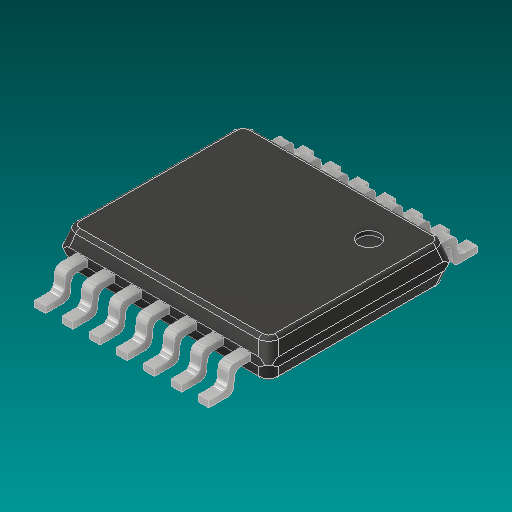
# Autodesk Inventor part: TSSOP
Saved by Autodesk Inventor 2017 (Build 210142000, 142)
## iProperties
Created: 2016-07-25
Part Number: TSSOP
Material: Generic
Document SubType Name: Modeling
Designer: Jonathan
Density: 1 g/cm^3
Appearance: Default
Author: Jonathan
Autodesk Inventor part; units mm, degrees
ref_plane "YZ Plane" through (0, 0, 0) normal (1, 0, 0) x (0, 1, 0)
ref_plane "XZ Plane" through (0, 0, 0) normal (0, 1, 0) x (-1, 0, 0)
ref_plane "XY Plane" through (0, 0, 0) normal (0, 0, 1) x (1, 0, 0)
sketch "Sketch1" plane through (0, 0, 0) normal (0, 1, 0) x (-1, 0, 0)
  line L0 (2.5, 2.2) -> (-2.5, 2.2)
  line L1 (-2.5, 2.2) -> (-2.5, -2.2)
  line L2 (-2.5, -2.2) -> (2.5, -2.2)
  line L3 (2.5, -2.2) -> (2.5, 2.2)
  line L4 (2.5, 2.2) -> (-2.5, -2.2) construction
  line L5 (-2.5, 2.2) -> (2.5, -2.2) construction
  point P0 (0, 0)
  dimension "d0" = 5
  dimension "d1" = 4.4
  constraints: 12 end point, 2 midpoint, 2 parallel, 1 horizontal, 1 perpendicular
  measures "d0" distance of L1.end L2.end
  measures "d1" distance of L0.end L1.end
extrude "Extrusion1" add sketch "Sketch1" along normal blind 0.9
sketch "Sketch3" plane through (0, 0, 0) normal (1, 0, 0) x (0, 1, 0)
  line L0 (0, 2.2) -> (0.9, 2.2) projected
  line L1 (0.525, 2.2) -> (0.525, 2.7167)
  line L2 (0.525, 2.7167) -> (0.05, 2.7582)
  line L3 (0.05, 2.7582) -> (0.05, 3.2)
  line L4 (0.05, 3.2) -> (-0.1, 3.2)
  line L5 (-0.1, 3.2) -> (-0.1, 2.6208)
  line L6 (-0.1, 2.6208) -> (0.375, 2.5792)
  line L7 (0.375, 2.5792) -> (0.375, 2.2)
  line L8 (0.525, 2.2) -> (0.375, 2.2)
  line L9 (0, 2.2) -> (0, -2.2) projected
  point P0 (0, 0)
  point P1 (0.1375, 2.6)
  point P2 (0.45, 2.2)
  dimension "d4" = 0.15
  dimension "d5" = 0.15
  dimension "d6" = 0.15
  dimension "d7" = 0.6
  dimension "d8" = 3.2
  dimension "d10" = 0.1
  dimension "d11" = 95
  constraints: 16 end point, 3 midpoint, 3 parallel, 2 perpendicular, 2 point on line, 1 collinear, 1 vertical
  measures "d4" distance between parallel lines of L5 L3
  measures "d5" distance between parallel lines of L2 L6
  measures "d6" distance between parallel lines of L1 L7
  measures "d7" distance from line of L4 point (0.138, 2.6)
  measures "d8" distance from line of point (0, 0) L4
  measures "d10" distance between parallel lines of L5 L9
  measures "d11" angle of L6 L5
extrude "Extrusion2" add sketch "Sketch3" along normal mid plane 0.25 separate body
fillet "Fillet1" radius 0.15 4 edges at (0, 0.05, 2.7582) (0, 0.525, 2.7167) (0, 0.375, 2.5792) (0, -0.1, 2.6208)
pattern_linear "Rectangular Pattern1" count 4 spacing 0.65 along (1, 0, 0) count 4 spacing 0.65 along (-1, 0, 0) of "Extrusion2", "Fillet1" bodies 2
mirror "Mirror1" about plane through (0, 0, 0) normal (0, 0, 1) of "Extrusion2", "Fillet1", "Rectangular Pattern1" bodies 2
chamfer "Chamfer1" distance 0.1 distance2 0.35 1 edges at (0, 0.9, 2.2) measured on face at (0.8333, 0.9, -0.7333)
chamfer "Chamfer2" distance 0.1 distance2 0.35 1 edges at (0, 0.9, -2.2) measured on face at (0.8333, 0.9, -0.7667)
chamfer "Chamfer3" distance 0.1 distance2 0.35 1 edges at (2.5, 0.9, 0) measured on face at (0.8333, 0.9, -0.7)
chamfer "Chamfer4" distance 0.1 distance2 0.35 1 edges at (-2.5, 0.9, 0) measured on face at (-0.8667, 0.9, -0.7)
chamfer "Chamfer5" distance 0.35 distance2 0.1 1 edges at (0, 0, 2.2) measured on face at (0.8333, 0.3667, 2.2)
chamfer "Chamfer6" distance 0.35 distance2 0.1 1 edges at (2.5, 0, -0.05) measured on face at (2.5, 0.3667, 0.7)
chamfer "Chamfer7" distance 0.35 distance2 0.1 1 edges at (-0.05, 0, -2.2) measured on face at (0.8, 0.3667, -2.2)
chamfer "Chamfer8" distance 0.35 distance2 0.1 1 edges at (-2.5, 0, 0) measured on face at (-2.5, 0.3667, 0.7)
fillet "Fillet2" radius 0.25 8 edges at (2.45, 0.725, 2.15) (2.45, 0.175, 2.15) (2.45, 0.725, -2.15) (2.45, 0.175, -2.15) (-2.45, 0.725, -2.15) (-2.45, 0.175, -2.15) (-2.45, 0.725, 2.15) (-2.45, 0.175, 2.15)
fillet "Fillet3" radius 0.1 16 edges at (-2.3307, 0.9, -2.0307) (0, 0.9, -2.1) (2.3307, 0.9, -2.0307) (2.4, 0.9, 0) (2.3307, 0.9, 2.0307) (0, 0.9, 2.1) (-2.3307, 0.9, 2.0307) (-2.4, 0.9, 0) (-2.3307, 0, 2.0307) (0, 0, 2.1) (2.3307, 0, 2.0307) (2.4, 0, 0) (2.3307, 0, -2.0307) (0, 0, -2.1) (-2.3307, 0, -2.0307) (-2.4, 0, 0)
sketch "Sketch4" plane through (0, 0.9, 0) normal (0, 1, 0) x (1, 0, 0)
  circle A0 centre (1.5, 1.2) radius 0.25
  line L0 (2.5, -1.9596) -> (2.5, 1.9596) projected
  line L1 (2.2596, 2.2) -> (-2.2596, 2.2) projected
  point P0 (0, 0)
  dimension "d47" = 0.5
  dimension "d48" = 1
  dimension "d49" = 1
  constraints: 1 centre point
  measures "d47" diameter of A0
  measures "d48" distance from line of L0 A0.centre
  measures "d49" distance from line of L1 A0.centre
extrude "Extrusion3" cut sketch "Sketch4" against normal blind 0.1 bodies 1
body "Solid1"
body "Solid2"
